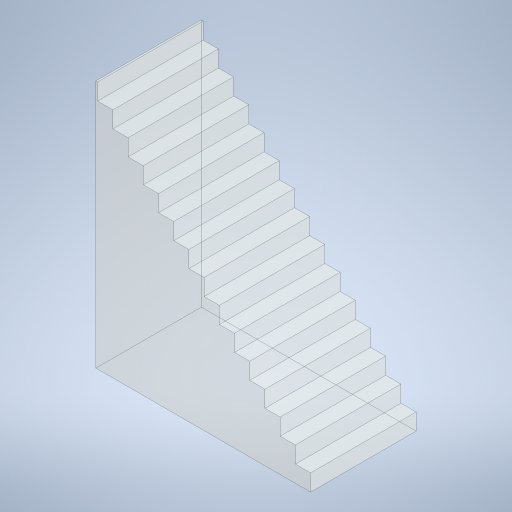
# Autodesk Inventor part: Stairs_Between_Finished_Basement_And_First_Floor
Saved by Autodesk Inventor 2024 (Build 280153000, 153)
## iProperties
Created: 2023-05-16
Part Number: Stairs_Between_Finished_Basement_And_First_Floor
Material: Steel
Document SubType Name: Modeling
Designer: Tom
Density: 7.85 g/cm^3
Appearance: Clear
Mass: 2.17052e+07 g
Surface Area: 147038 cm^2
Volume: 2.765e+06 cm^3
Author: Tom
Autodesk Inventor part; units mm, degrees
ref_plane "YZ Plane" through (0, 0, 0) normal (1, 0, 0) x (0, 1, 0)
ref_plane "XZ Plane" through (0, 0, 0) normal (0, 1, 0) x (-1, 0, 0)
ref_plane "XY Plane" through (0, 0, 0) normal (0, 0, 1) x (1, 0, 0)
sketch "Sketch1" plane through (0, 0, 0) normal (0, 0, 1) x (1, 0, 0)
  line L0 (-161.925, 176.53) -> (-161.925, 353.06)
  line L1 (-161.925, 353.06) -> (-323.85, 353.06)
  line L2 (-323.85, 353.06) -> (-323.85, 529.59)
  line L3 (-323.85, 529.59) -> (-485.775, 529.59)
  line L4 (-485.775, 529.59) -> (-485.775, 706.12)
  line L5 (-485.775, 706.12) -> (-647.7, 706.12)
  line L6 (-647.7, 706.12) -> (-647.7, 882.65)
  line L7 (-647.7, 882.65) -> (-809.625, 882.65)
  line L8 (-809.625, 882.65) -> (-809.625, 1059.18)
  line L9 (-809.625, 1059.18) -> (-971.55, 1059.18)
  line L10 (-971.55, 1059.18) -> (-971.55, 1235.71)
  line L11 (-971.55, 1235.71) -> (-1133.475, 1235.71)
  line L12 (-1133.475, 1235.71) -> (-1133.475, 1412.24)
  line L13 (-1133.475, 1412.24) -> (-1295.4, 1412.24)
  line L14 (-1295.4, 1412.24) -> (-1295.4, 1588.77)
  line L15 (-1295.4, 1588.77) -> (-1457.325, 1588.77)
  line L16 (-1457.325, 1588.77) -> (-1457.325, 1765.3)
  line L17 (-1457.325, 1765.3) -> (-1619.25, 1765.3)
  line L18 (-1619.25, 1765.3) -> (-1619.25, 1941.83)
  line L19 (-1619.25, 1941.83) -> (-1781.175, 1941.83)
  line L20 (-1781.175, 1941.83) -> (-1781.175, 2118.36)
  line L21 (-1781.175, 2118.36) -> (-1943.1, 2118.36)
  line L22 (-1943.1, 2118.36) -> (-1943.1, 2294.89)
  line L23 (-1943.1, 2294.89) -> (-2105.025, 2294.89)
  line L24 (-161.925, 176.53) -> (0, 176.53)
  line L25 (0, 176.53) -> (0, 0)
  line L26 (0, 0) -> (-2286, 0)
  line L27 (-2105.025, 2294.89) -> (-2105.025, 2471.42)
  line L28 (-2105.025, 2471.42) -> (-2266.95, 2471.42)
  line L29 (-2266.95, 2471.42) -> (-2266.95, 2647.95)
  line L30 (-2266.95, 2647.95) -> (-2286, 2647.95)
  line L31 (-2286, 2647.95) -> (-2286, 0)
  point P0 (-2762.8302, 625.5305)
  dimension "d21" = 2647.95
  dimension "d22" = 2286
  dimension "d23" = 19.05
  constraints: 64 end point, 27 parallel, 26 perpendicular, 3 horizontal, 3 vertical, 1 coincident
  measures "d21" distance of L30.end L26.end
  measures "d22" distance of L25.end L26.end
  measures "d23" distance of L29.end L30.end
extrude "Extrusion1" add sketch "Sketch1" along normal blind 1123.95
body "Solid1"
